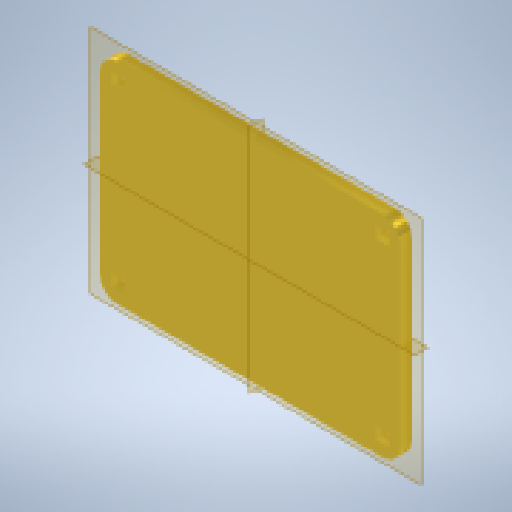
# Autodesk Inventor part: Sessao8_07_04_2025_0001_0001
Saved by Autodesk Inventor 2025.2 (Build 292293000, 293)
## iProperties
Created: 2025-04-07
Part Number: Sessao8_07_04_2025_0001_0001
Material: Ouro
Document SubType Name: Modeling
Designer: Gustavo Sousa
Density: 19.3 g/cm^3
Appearance: Metal quente 2400F
Author: Gustavo Sousa
Autodesk Inventor part; units mm, degrees
sketch "Esboço1" plane through (0, 0, 0) normal (0, 0, 1) x (1, 0, 0)
  line L0 (-250, -175) -> (250, -175)
  line L1 (250, -175) -> (250, 175)
  line L2 (250, 175) -> (-250, 175)
  line L3 (-250, 175) -> (-250, -175)
  line L4 (-250, -175) -> (250, 175) construction
  line L5 (250, -175) -> (-250, 175) construction
  point P0 (0, 0)
  dimension "d0" = 500
  dimension "d1" = 350
  constraints: 12 end point, 2 midpoint, 2 parallel, 1 horizontal, 1 perpendicular
  measures "d0" distance of L2.end L1.end
  measures "d1" distance of L1.end L0.end
extrude "Extrusão1" add sketch "Esboço1" along normal mid plane 20
fillet "Arredondamento1" radius 30 4 edges at (-250, 175, 0) (250, 175, 0) (250, -175, 0) (-250, -175, 0)
sketch "Esboço2" plane through (0, 0, 10) normal (0, 0, 1) x (1, 0, 0)
  line L0 (230, 135) -> (230, 155) projected
  line L1 (230, 155) -> (210, 155) projected
  line L2 (210, 155) -> (210, 135) projected
  line L3 (210, 135) -> (230, 135) projected
  line L4 (212, 137) -> (212, 153) projected
  line L5 (212, 153) -> (228, 153) projected
  line L6 (228, 153) -> (228, 137) projected
  line L7 (228, 137) -> (212, 137) projected
  line L8 (209.8, 155.2) -> (230.2, 155.2)
  line L9 (230.2, 155.2) -> (230.2, 134.8)
  line L10 (230.2, 134.8) -> (209.8, 134.8)
  line L11 (209.8, 134.8) -> (209.8, 155.2)
  line L12 (-210, 135) -> (-210, 155) projected
  line L13 (-210, 155) -> (-230, 155) projected
  line L14 (-230, 155) -> (-230, 135) projected
  line L15 (-230, 135) -> (-210, 135) projected
  line L16 (-228, 137) -> (-228, 153) projected
  line L17 (-228, 153) -> (-212, 153) projected
  line L18 (-212, 153) -> (-212, 137) projected
  line L19 (-212, 137) -> (-228, 137) projected
  line L20 (-210, -155) -> (-210, -135) projected
  line L21 (-210, -135) -> (-230, -135) projected
  line L22 (-230, -135) -> (-230, -155) projected
  line L23 (-230, -155) -> (-210, -155) projected
  line L24 (-228, -153) -> (-228, -137) projected
  line L25 (-228, -137) -> (-212, -137) projected
  line L26 (-212, -137) -> (-212, -153) projected
  line L27 (-212, -153) -> (-228, -153) projected
  line L28 (230, -135) -> (230, -155) projected
  line L29 (230, -155) -> (210, -155) projected
  line L30 (210, -155) -> (210, -135) projected
  line L31 (210, -135) -> (230, -135) projected
  line L32 (212, -137) -> (212, -153) projected
  line L33 (212, -153) -> (228, -153) projected
  line L34 (228, -153) -> (228, -137) projected
  line L35 (228, -137) -> (212, -137) projected
  line L36 (-230.2, 155.2) -> (-209.8, 155.2)
  line L37 (-209.8, 155.2) -> (-209.8, 134.8)
  line L38 (-209.8, 134.8) -> (-230.2, 134.8)
  line L39 (-230.2, 134.8) -> (-230.2, 155.2)
  line L40 (-230.2, -134.8) -> (-209.8, -134.8)
  line L41 (-209.8, -134.8) -> (-209.8, -155.2)
  line L42 (-209.8, -155.2) -> (-230.2, -155.2)
  line L43 (-230.2, -155.2) -> (-230.2, -134.8)
  line L44 (230.2, -155.2) -> (230.2, -134.8)
  line L45 (230.2, -134.8) -> (209.8, -134.8)
  line L46 (209.8, -134.8) -> (209.8, -155.2)
  line L47 (209.8, -155.2) -> (230.2, -155.2)
  point P0 (0, 0)
  dimension "d5" = 0.2
  dimension "d6" = 0.2
  dimension "d7" = 0.2
  dimension "d8" = 0.2
  constraints: 32 end point, 12 other
  measures "d5" distance between parallel lines of L1 L8
  measures "d6" distance between parallel lines of L13 L36
  measures "d7" distance between parallel lines of L21 L40
  measures "d8" distance between parallel lines of L31 L45
extrude "Extrusão2" cut sketch "Esboço2" against normal blind 20 contours L3 L2 L1 L0 | L4 L5 L6 L7 | L8 L9 L10 L11 | L15 L14 L13 L12 | L16 L17 L18 L19 | L23 L22 L21 L20 | L24 L25 L26 L27 | L28 L29 L30 L31 | L35 L34 L33 L32 | L36 L37 L38 L39 | L40 L41 L42 L43 | L47 L46 L45 L44
